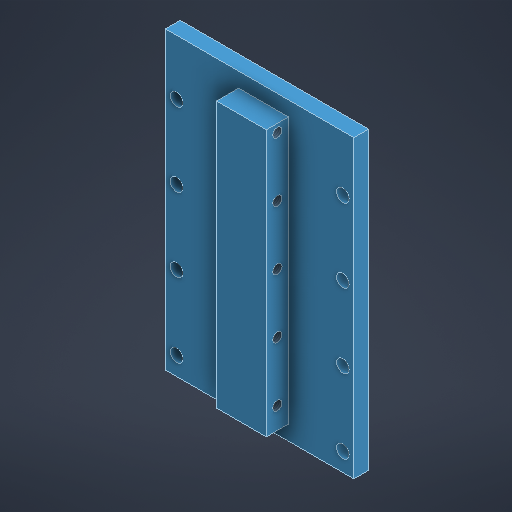
# Autodesk Inventor part: Rod_Holder_Adapter
Saved by Autodesk Inventor 2027.1 (Build 311270010, 270A)
## iProperties
Created: 2026-09-21
Part Number: Rod_Holder_Adapter
Material: Generic
Document SubType Name: Modeling
Designer: 박정현
Density: 1 g/cm^3
Appearance: New hanging adapter - material unassigned
Author: 박정현
Comments: 80 mm solid plate matching the 79.44 mm device length, with integral raised mounting boss. Both opposite boss faces have five right-hand M3 x 0.5 - 6H internal threads at 16 mm pitch, 10 total. Native cosmetic thread features; 6 mm depth per side, 1.5 mm solid web between opposed bores. Existing Top_ForFridge slots and source parts unchanged.
Autodesk Inventor part; units mm, degrees
sketch "Continuous_Solid_Plate_No_Openings_Profile" plane through (0, 0, 0) normal (0, 0, 1) x (1, 0, 0)
  line L0 (0, 0) -> (51, 0)
  line L1 (51, 0) -> (51, 80)
  line L2 (51, 80) -> (0, 80)
  line L3 (0, 80) -> (0, 0)
  dimension "d0" = 51
  dimension "d1" = 80
  constraints: 8 end point, 2 parallel, 1 coincident, 1 horizontal, 1 perpendicular
  measures "d0" distance of L1.end L2.end
  measures "d1" distance of L2.end L0.start
extrude "Continuous_Solid_Plate_No_Openings" add sketch "Continuous_Solid_Plate_No_Openings_Profile" along normal blind 4
ref_plane "Integral_Raised_Device_Mounting_Boss_StartPlane" through (0, 0, 4) normal (0, 0, 1) x (1, 0, 0)
sketch "Integral_Raised_Device_Mounting_Boss_Profile" plane through (0, 0, 4) normal (0, 0, 1) x (1, 0, 0)
  line L0 (19.7942, 4) -> (33.2942, 4)
  line L1 (33.2942, 4) -> (33.2942, 76)
  line L2 (33.2942, 76) -> (19.7942, 76)
  line L3 (19.7942, 76) -> (19.7942, 4)
  point P0 (0, 0)
  dimension "d5" = 19.7943
  dimension "d6" = 4
  dimension "d7" = 13.5
  dimension "d8" = 72
  constraints: 8 end point, 2 parallel, 1 horizontal, 1 perpendicular
  measures "d5" horizontal distance of point (0, 0) L0.start
  measures "d6" vertical distance of point (0, 0) L0.start
  measures "d7" distance of L1.end L2.end
  measures "d8" distance of L2.end L0.start
extrude "Integral_Raised_Device_Mounting_Boss" add sketch "Integral_Raised_Device_Mounting_Boss_Profile" along normal blind 6
sketch "Rod_M3_Clearance_8x_Locations" plane through (0, 0, 0) normal (0, 0, 1) x (1, 0, 0)
  circle A0 centre (3, 5) radius 1.7
  circle A1 centre (3, 25) radius 1.7
  circle A2 centre (3, 45) radius 1.7
  circle A3 centre (3, 65) radius 1.7
  circle A4 centre (48, 5) radius 1.7
  circle A5 centre (48, 25) radius 1.7
  circle A6 centre (48, 45) radius 1.7
  circle A7 centre (48, 65) radius 1.7
  point P0 (0, 0)
  dimension "d11" = 3
  dimension "d12" = 5
  dimension "d13" = 3.4
  dimension "d14" = 3
  dimension "d15" = 25
  dimension "d16" = 3.4
  dimension "d17" = 3
  dimension "d18" = 45
  dimension "d19" = 3.4
  dimension "d20" = 3
  dimension "d21" = 65
  dimension "d22" = 3.4
  dimension "d23" = 48
  dimension "d24" = 5
  dimension "d25" = 3.4
  dimension "d26" = 48
  dimension "d27" = 25
  dimension "d28" = 3.4
  dimension "d29" = 48
  dimension "d30" = 45
  dimension "d31" = 3.4
  dimension "d32" = 48
  dimension "d33" = 65
  dimension "d34" = 3.4
  constraints: 8 centre point
  measures "d11" horizontal distance of point (0, 0) A0.centre
  measures "d12" vertical distance of point (0, 0) A0.centre
  measures "d13" diameter of A0
  measures "d14" horizontal distance of point (0, 0) A1.centre
  measures "d15" vertical distance of point (0, 0) A1.centre
  measures "d16" diameter of A1
  measures "d17" horizontal distance of point (0, 0) A2.centre
  measures "d18" vertical distance of point (0, 0) A2.centre
  measures "d19" diameter of A2
  measures "d20" horizontal distance of point (0, 0) A3.centre
  measures "d21" vertical distance of point (0, 0) A3.centre
  measures "d22" diameter of A3
  measures "d23" horizontal distance of point (0, 0) A4.centre
  measures "d24" vertical distance of point (0, 0) A4.centre
  measures "d25" diameter of A4
  measures "d26" horizontal distance of point (0, 0) A5.centre
  measures "d27" vertical distance of point (0, 0) A5.centre
  measures "d28" diameter of A5
  measures "d29" horizontal distance of point (0, 0) A6.centre
  measures "d30" vertical distance of point (0, 0) A6.centre
  measures "d31" diameter of A6
  measures "d32" horizontal distance of point (0, 0) A7.centre
  measures "d33" vertical distance of point (0, 0) A7.centre
  measures "d34" diameter of A7
extrude "Rod_M3_Clearance_8x" cut sketch "Rod_M3_Clearance_8x_Locations" along normal through all
ref_plane "Device_Clamp_Face_PositiveX" through (33.2942, 0, 0) normal (1, 0, 0) x (0, 1, 0)
sketch "M3_Side_Tap_Locations_PositiveX" plane through (33.2942, 0, 0) normal (1, 0, 0) x (0, 1, 0)
  circle A0 centre (9.828, 7) radius 1.25
  circle A1 centre (25.828, 7) radius 1.25
  circle A2 centre (41.828, 7) radius 1.25
  circle A3 centre (57.828, 7) radius 1.25
  circle A4 centre (73.828, 7) radius 1.25
  point P0 (0, 0)
  dimension "d38" = 9.828
  dimension "d39" = 7
  dimension "d40" = 2.5
  dimension "d41" = 25.828
  dimension "d42" = 7
  dimension "d43" = 2.5
  dimension "d44" = 41.828
  dimension "d45" = 7
  dimension "d46" = 2.5
  dimension "d47" = 57.828
  dimension "d48" = 7
  dimension "d49" = 2.5
  dimension "d50" = 73.828
  dimension "d51" = 7
  dimension "d52" = 2.5
  constraints: 5 centre point
  measures "d38" horizontal distance of point (0, 0) A0.centre
  measures "d39" vertical distance of point (0, 0) A0.centre
  measures "d40" diameter of A0
  measures "d41" horizontal distance of point (0, 0) A1.centre
  measures "d42" vertical distance of point (0, 0) A1.centre
  measures "d43" diameter of A1
  measures "d44" horizontal distance of point (0, 0) A2.centre
  measures "d45" vertical distance of point (0, 0) A2.centre
  measures "d46" diameter of A2
  measures "d47" horizontal distance of point (0, 0) A3.centre
  measures "d48" vertical distance of point (0, 0) A3.centre
  measures "d49" diameter of A3
  measures "d50" horizontal distance of point (0, 0) A4.centre
  measures "d51" vertical distance of point (0, 0) A4.centre
  measures "d52" diameter of A4
extrude "Device_Tap_Drills_5x_PositiveX" cut sketch "M3_Side_Tap_Locations_PositiveX" against normal blind 6
thread "Device_M3x0_5_6H_PositiveX_1" size "M3x0.5" class "6H" standard "ISO Metric profile" length 6
thread "Device_M3x0_5_6H_PositiveX_2" size "M3x0.5" class "6H" standard "ISO Metric profile" length 6
thread "Device_M3x0_5_6H_PositiveX_3" size "M3x0.5" class "6H" standard "ISO Metric profile" length 6
thread "Device_M3x0_5_6H_PositiveX_4" size "M3x0.5" class "6H" standard "ISO Metric profile" length 6
thread "Device_M3x0_5_6H_PositiveX_5" size "M3x0.5" class "6H" standard "ISO Metric profile" length 6
ref_plane "Device_Clamp_Face_NegativeX" through (19.7942, 0, 0) normal (1, 0, 0) x (0, 1, 0)
sketch "M3_Side_Tap_Locations_NegativeX" plane through (19.7942, 0, 0) normal (1, 0, 0) x (0, 1, 0)
  circle A0 centre (9.828, 7) radius 1.25
  circle A1 centre (25.828, 7) radius 1.25
  circle A2 centre (41.828, 7) radius 1.25
  circle A3 centre (57.828, 7) radius 1.25
  circle A4 centre (73.828, 7) radius 1.25
  point P0 (0, 0)
  dimension "d66" = 9.828
  dimension "d67" = 7
  dimension "d68" = 2.5
  dimension "d69" = 25.828
  dimension "d70" = 7
  dimension "d71" = 2.5
  dimension "d72" = 41.828
  dimension "d73" = 7
  dimension "d74" = 2.5
  dimension "d75" = 57.828
  dimension "d76" = 7
  dimension "d77" = 2.5
  dimension "d78" = 73.828
  dimension "d79" = 7
  dimension "d80" = 2.5
  constraints: 5 centre point
  measures "d66" horizontal distance of point (0, 0) A0.centre
  measures "d67" vertical distance of point (0, 0) A0.centre
  measures "d68" diameter of A0
  measures "d69" horizontal distance of point (0, 0) A1.centre
  measures "d70" vertical distance of point (0, 0) A1.centre
  measures "d71" diameter of A1
  measures "d72" horizontal distance of point (0, 0) A2.centre
  measures "d73" vertical distance of point (0, 0) A2.centre
  measures "d74" diameter of A2
  measures "d75" horizontal distance of point (0, 0) A3.centre
  measures "d76" vertical distance of point (0, 0) A3.centre
  measures "d77" diameter of A3
  measures "d78" horizontal distance of point (0, 0) A4.centre
  measures "d79" vertical distance of point (0, 0) A4.centre
  measures "d80" diameter of A4
extrude "Device_Tap_Drills_5x_NegativeX" cut sketch "M3_Side_Tap_Locations_NegativeX" along normal blind 6
thread "Device_M3x0_5_6H_NegativeX_1" size "M3x0.5" class "6H" standard "ISO Metric profile" length 6
thread "Device_M3x0_5_6H_NegativeX_2" size "M3x0.5" class "6H" standard "ISO Metric profile" length 6
thread "Device_M3x0_5_6H_NegativeX_3" size "M3x0.5" class "6H" standard "ISO Metric profile" length 6
thread "Device_M3x0_5_6H_NegativeX_4" size "M3x0.5" class "6H" standard "ISO Metric profile" length 6
thread "Device_M3x0_5_6H_NegativeX_5" size "M3x0.5" class "6H" standard "ISO Metric profile" length 6
equation "\"d0\" = OverallWidth"
equation "\"d1\" = ContactLength"
equation "\"d2\" = BaseThickness"
equation "\"d5\" = FingerStartX"
equation "\"d6\" = FingerEndInset"
equation "\"d7\" = FingerWidth"
equation "\"d8\" = ContactLength - 2 * FingerEndInset"
equation "\"d9\" = FingerThickness"
equation "\"d11\" = 0.5 * RodWidth"
equation "\"d12\" = RodHoleStart + 0 * RodScrewPitch"
equation "\"d13\" = RodClearanceDiameter"
equation "\"d14\" = 0.5 * RodWidth"
equation "\"d15\" = RodHoleStart + RodScrewPitch"
equation "\"d16\" = RodClearanceDiameter"
equation "\"d17\" = 0.5 * RodWidth"
equation "\"d18\" = RodHoleStart + 2 * RodScrewPitch"
equation "\"d19\" = RodClearanceDiameter"
equation "\"d20\" = 0.5 * RodWidth"
equation "\"d21\" = RodHoleStart + 3 * RodScrewPitch"
equation "\"d22\" = RodClearanceDiameter"
equation "\"d23\" = OverallWidth - 0.5 * RodWidth"
equation "\"d24\" = RodHoleStart + 0 * RodScrewPitch"
equation "\"d25\" = RodClearanceDiameter"
equation "\"d26\" = OverallWidth - 0.5 * RodWidth"
equation "\"d27\" = RodHoleStart + RodScrewPitch"
equation "\"d28\" = RodClearanceDiameter"
equation "\"d29\" = OverallWidth - 0.5 * RodWidth"
equation "\"d30\" = RodHoleStart + 2 * RodScrewPitch"
equation "\"d31\" = RodClearanceDiameter"
equation "\"d32\" = OverallWidth - 0.5 * RodWidth"
equation "\"d33\" = RodHoleStart + 3 * RodScrewPitch"
equation "\"d34\" = RodClearanceDiameter"
equation "\"d38\" = ClampFirstY - 2 * ClampPitch"
equation "\"d39\" = ClampHeight"
equation "\"d40\" = TapDrillDiameter"
equation "\"d41\" = ClampFirstY - ClampPitch"
equation "\"d42\" = ClampHeight"
equation "\"d43\" = TapDrillDiameter"
equation "\"d44\" = ClampFirstY + 0 * ClampPitch"
equation "\"d45\" = ClampHeight"
equation "\"d46\" = TapDrillDiameter"
equation "\"d47\" = ClampFirstY + ClampPitch"
equation "\"d48\" = ClampHeight"
equation "\"d49\" = TapDrillDiameter"
equation "\"d50\" = ClampFirstY + 2 * ClampPitch"
equation "\"d51\" = ClampHeight"
equation "\"d52\" = TapDrillDiameter"
equation "\"d53\" = TapDepth"
equation "\"d55\" = TapDepth"
equation "\"d57\" = TapDepth"
equation "\"d59\" = TapDepth"
equation "\"d61\" = TapDepth"
equation "\"d63\" = TapDepth"
equation "\"d66\" = ClampFirstY - 2 * ClampPitch"
equation "\"d67\" = ClampHeight"
equation "\"d68\" = TapDrillDiameter"
equation "\"d69\" = ClampFirstY - ClampPitch"
equation "\"d70\" = ClampHeight"
equation "\"d71\" = TapDrillDiameter"
equation "\"d72\" = ClampFirstY + 0 * ClampPitch"
equation "\"d73\" = ClampHeight"
equation "\"d74\" = TapDrillDiameter"
equation "\"d75\" = ClampFirstY + ClampPitch"
equation "\"d76\" = ClampHeight"
equation "\"d77\" = TapDrillDiameter"
equation "\"d78\" = ClampFirstY + 2 * ClampPitch"
equation "\"d79\" = ClampHeight"
equation "\"d80\" = TapDrillDiameter"
equation "\"d81\" = TapDepth"
equation "\"d83\" = TapDepth"
equation "\"d85\" = TapDepth"
equation "\"d87\" = TapDepth"
equation "\"d89\" = TapDepth"
equation "\"d91\" = TapDepth"
equation "\"OverallWidth\" = 51"
equation "\"RodWidth\" = 6"
equation "\"ContactLength\" = 80"
equation "\"BaseThickness\" = 4"
equation "\"FingerStartX\" = 19.79425"
equation "\"FingerWidth\" = 13.5"
equation "\"FingerThickness\" = 6"
equation "\"FingerEndInset\" = 4"
equation "\"RodClearanceDiameter\" = 3.4"
equation "\"ClampFirstY\" = 41.82802"
equation "\"ClampPitch\" = 16"
equation "\"ClampHeight\" = 7"
equation "\"TapDrillDiameter\" = 2.5"
equation "\"TapDepth\" = 6"
equation "\"RodHoleStart\" = 5"
equation "\"RodScrewPitch\" = 20"
equation "\"d4\" = BaseThickness"
equation "\"d37\" = FingerStartX + FingerWidth"
equation "\"d65\" = FingerStartX"
body "Solid1"
